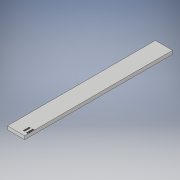
# Autodesk Inventor part: HDI
Saved by Autodesk Inventor 2019.4 (Build 234330000, 330)
## iProperties
Created: 2021-02-08
Part Number: HDI
Material: Generic
Document SubType Name: Modeling
Designer: caleb
Density: 1 g/cm^3
Appearance: Default
Author: caleb
Autodesk Inventor part; units mm, degrees
ref_plane "YZ Plane" through (0, 0, 0) normal (1, 0, 0) x (0, 1, 0)
ref_plane "XZ Plane" through (0, 0, 0) normal (0, 1, 0) x (-1, 0, 0)
ref_plane "XY Plane" through (0, 0, 0) normal (0, 0, 1) x (1, 0, 0)
sketch "Sketch1" plane through (0, 0, 0) normal (0, 1, 0) x (-1, 0, 0)
  line L0 (-2.5, 21.5) -> (2.5, 21.5)
  line L1 (2.5, 21.5) -> (2.5, -21.5)
  line L2 (2.5, -21.5) -> (-2.5, -21.5)
  line L3 (-2.5, -21.5) -> (-2.5, 21.5)
  line L4 (-2.5, 21.5) -> (2.5, -21.5) construction
  line L5 (2.5, 21.5) -> (-2.5, -21.5) construction
  point P0 (0, 0)
  dimension "d0" = 43
  dimension "d1" = 5
  constraints: 12 end point, 2 midpoint, 2 parallel, 1 horizontal, 1 perpendicular
  measures "d0" distance of L0.end L1.end
  measures "d1" distance of L0.start L0.end
extrude "Extrusion1" add sketch "Sketch1" along normal blind 1
sketch "Sketch2" plane through (0, 1, 0) normal (0, 1, 0) x (1, 0, 0)
  line L0 (2, -20.5) -> (2.4, -20.5)
  line L1 (2.4, -20.5) -> (2.4, -20.4)
  line L2 (2.4, -20.4) -> (2, -20.4)
  line L3 (2, -20.4) -> (2, -20.5)
  line L4 (2, -20.5) -> (2.4, -20.4) construction
  line L5 (2.4, -20.5) -> (2, -20.4) construction
  line L6 (2.5, -21.5) -> (2.5, 21.5) projected
  line L7 (-2.5, -21.5) -> (2.5, -21.5) projected
  line L8 (2.4, -20.3) -> (2.4, -20.2)
  line L9 (2.4, -20.2) -> (2, -20.2)
  line L10 (2, -20.2) -> (2, -20.3)
  line L11 (2, -20.3) -> (2.4, -20.3)
  line L12 (2.4, -20.1) -> (2.4, -20)
  line L13 (2.4, -20) -> (2, -20)
  line L14 (2, -20) -> (2, -20.1)
  line L15 (2, -20.1) -> (2.4, -20.1)
  line L16 (2.4, -19.9) -> (2.4, -19.8)
  line L17 (2.4, -19.8) -> (2, -19.8)
  line L18 (2, -19.8) -> (2, -19.9)
  line L19 (2, -19.9) -> (2.4, -19.9)
  line L20 (2.4, -19.7) -> (2.4, -19.6)
  line L21 (2.4, -19.6) -> (2, -19.6)
  line L22 (2, -19.6) -> (2, -19.7)
  line L23 (2, -19.7) -> (2.4, -19.7)
  line L24 (2.4, -19.5) -> (2.4, -19.4)
  line L25 (2.4, -19.4) -> (2, -19.4)
  line L26 (2, -19.4) -> (2, -19.5)
  line L27 (2, -19.5) -> (2.4, -19.5)
  line L28 (2.4, -19.3) -> (2.4, -19.2)
  line L29 (2.4, -19.2) -> (2, -19.2)
  line L30 (2, -19.2) -> (2, -19.3)
  line L31 (2, -19.3) -> (2.4, -19.3)
  line L32 (2.4, -19.1) -> (2.4, -19)
  line L33 (2.4, -19) -> (2, -19)
  line L34 (2, -19) -> (2, -19.1)
  line L35 (2, -19.1) -> (2.4, -19.1)
  line L36 (2.4, -18.9) -> (2.4, -18.8)
  line L37 (2.4, -18.8) -> (2, -18.8)
  line L38 (2, -18.8) -> (2, -18.9)
  line L39 (2, -18.9) -> (2.4, -18.9)
  line L40 (2.4, -18.7) -> (2.4, -18.6)
  line L41 (2.4, -18.6) -> (2, -18.6)
  line L42 (2, -18.6) -> (2, -18.7)
  line L43 (2, -18.7) -> (2.4, -18.7)
  line L44 (1, -20.4) -> (1.4, -20.4)
  line L45 (1.4, -20.4) -> (1.4, -20.3)
  line L46 (1.4, -20.3) -> (1, -20.3)
  line L47 (1, -20.3) -> (1, -20.4)
  line L48 (1, -20.4) -> (1.4, -20.3) construction
  line L49 (1.4, -20.4) -> (1, -20.3) construction
  line L50 (1.4, -20.1) -> (1, -20.1)
  line L51 (1, -20.2) -> (1.4, -20.2)
  line L52 (1, -20.1) -> (1, -20.2)
  line L53 (1, -20.2) -> (1.4, -20.1) construction
  line L54 (1.4, -20.2) -> (1, -20.1) construction
  line L55 (1.4, -20.2) -> (1.4, -20.1)
  line L56 (1.4, -19.9) -> (1, -19.9)
  line L57 (1, -20) -> (1.4, -20)
  line L58 (1, -19.9) -> (1, -20)
  line L59 (1, -20) -> (1.4, -19.9) construction
  line L60 (1.4, -20) -> (1, -19.9) construction
  line L61 (1.4, -20) -> (1.4, -19.9)
  line L62 (1.4, -19.7) -> (1, -19.7)
  line L63 (1, -19.8) -> (1.4, -19.8)
  line L64 (1, -19.7) -> (1, -19.8)
  line L65 (1, -19.8) -> (1.4, -19.7) construction
  line L66 (1.4, -19.8) -> (1, -19.7) construction
  line L67 (1.4, -19.8) -> (1.4, -19.7)
  line L68 (1.4, -19.5) -> (1, -19.5)
  line L69 (1, -19.6) -> (1.4, -19.6)
  line L70 (1, -19.5) -> (1, -19.6)
  line L71 (1, -19.6) -> (1.4, -19.5) construction
  line L72 (1.4, -19.6) -> (1, -19.5) construction
  line L73 (1.4, -19.6) -> (1.4, -19.5)
  line L74 (1.4, -19.3) -> (1, -19.3)
  line L75 (1, -19.4) -> (1.4, -19.4)
  line L76 (1, -19.3) -> (1, -19.4)
  line L77 (1, -19.4) -> (1.4, -19.3) construction
  line L78 (1.4, -19.4) -> (1, -19.3) construction
  line L79 (1.4, -19.4) -> (1.4, -19.3)
  line L80 (1.4, -19.1) -> (1, -19.1)
  line L81 (1, -19.2) -> (1.4, -19.2)
  line L82 (1, -19.1) -> (1, -19.2)
  line L83 (1, -19.2) -> (1.4, -19.1) construction
  line L84 (1.4, -19.2) -> (1, -19.1) construction
  line L85 (1.4, -19.2) -> (1.4, -19.1)
  line L86 (1.4, -18.9) -> (1, -18.9)
  line L87 (1, -19) -> (1.4, -19)
  line L88 (1, -18.9) -> (1, -19)
  line L89 (1, -19) -> (1.4, -18.9) construction
  line L90 (1.4, -19) -> (1, -18.9) construction
  line L91 (1.4, -19) -> (1.4, -18.9)
  line L92 (1.4, -18.7) -> (1, -18.7)
  line L93 (1, -18.8) -> (1.4, -18.8)
  line L94 (1, -18.7) -> (1, -18.8)
  line L95 (1, -18.8) -> (1.4, -18.7) construction
  line L96 (1.4, -18.8) -> (1, -18.7) construction
  line L97 (1.4, -18.8) -> (1.4, -18.7)
  point P0 (0, 0)
  point P1 (2.2, -20.45)
  point P2 (2.2, -20.25)
  point P3 (2.2, -20.05)
  point P4 (2.2, -19.85)
  point P5 (2.2, -19.65)
  point P6 (2.2, -19.45)
  point P7 (2.2, -19.25)
  point P8 (2.2, -19.05)
  point P9 (2.2, -18.85)
  point P10 (2.2, -18.65)
  point P11 (1.2, -20.35)
  point P12 (1.2, -20.15)
  point P13 (1.2, -19.95)
  point P14 (1.2, -19.75)
  point P15 (1.2, -19.55)
  point P16 (1.2, -19.35)
  point P17 (1.2, -19.15)
  point P18 (1.2, -18.95)
  point P19 (1.2, -18.75)
  dimension "d4" = 0.1
  dimension "d5" = 0.4
  dimension "d6" = 0.1
  dimension "d7" = 1
  dimension "d10" = 0.2
  dimension "d15" = 1.1
  dimension "d16" = 1
  dimension "d19" = 0.2
  constraints: 192 end point, 20 midpoint, 6 parallel, 2 horizontal, 2 perpendicular, 2 vertical, 169 other
  measures "d4" distance of L2.end L0.start
  measures "d5" distance of L1.end L2.end
  measures "d6" distance between parallel lines of L6 L1
  measures "d7" distance between parallel lines of L7 L0
  measures "d10" distance of L0.end L8.start
  measures "d15" distance between parallel lines of L7 L44
  measures "d16" distance between parallel lines of L45 L8
  measures "d19" distance of L45.end L50.start
extrude "Extrusion2" add sketch "Sketch2" along normal blind 0.03
body "Solid1"
